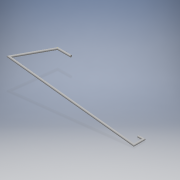
# Autodesk Inventor part: WIRE
Saved by Autodesk Inventor 2017 (Build 210142000, 142)
## iProperties
Created: 2017-12-26
Part Number: WIRE
Material: Generic
Document SubType Name: Modeling
Designer: will
Density: 1 g/cm^3
Appearance: Default
Author: will
Autodesk Inventor part; units mm, degrees
ref_plane "YZ Plane" through (0, 0, 0) normal (1, 0, 0) x (0, 1, 0)
ref_plane "XZ Plane" through (0, 0, 0) normal (0, 1, 0) x (-1, 0, 0)
ref_plane "XY Plane" through (0, 0, 0) normal (0, 0, 1) x (1, 0, 0)
sketch "Sketch1" plane through (0, 0, 0) normal (0, 0, 1) x (1, 0, 0)
  circle A0 centre (-10.0785, 9.8744) radius 0.8047
  point P0 (0, 0)
  constraints: 1 centre point
sketch3d "3D Sketch1"
  line L0 (-108.4342, 25.2423, -12.8177) -> (-113.0178, 25.2403, -13.7938)
  arc A0 (-113.0178, 25.2403, -13.7938) -> (-115.4344, 25.2393, -11.8377) centre (-113.4344, 25.2402, -11.8377) ccw
  line L1 (-115.4344, 25.2393, -11.8377) -> (-115.4344, 25.2393, 1.4693)
  arc A1 (-115.4344, 25.2393, 1.4693) -> (-113.4532, 24.9504, 3.4693) centre (-113.4554, 24.9507, 1.4693) ccw
  line L2 (-113.4532, 24.9504, 3.4693) -> (-12.0554, 10.1627, 3.3569)
  arc A2 (-12.0554, 10.1627, 3.3569) -> (-10.0785, 9.8744, 1.3569) centre (-12.0576, 10.163, 1.3569) ccw
  line L3 (-10.0785, 9.8744, 1.3569) -> (-10.0785, 9.8744, 0)
  line L4 (-10.0785, 9.8744, 0) -> (-10.0785, 9.8744, -2.8366)
  arc A3 (-10.0785, 9.8744, -2.8366) -> (-12.0785, 9.8744, -4.8366) centre (-12.0785, 9.8744, -2.8366) ccw
  line L5 (-12.0785, 9.8744, -4.8366) -> (-14.5001, 9.8744, -4.8366)
  dimension "d6" = 17.78
  dimension "d2" = 2
  dimension "d3" = 2
  dimension "d4" = 2
  dimension "d5" = 2
  constraints: 2 vertical, 6 other
sweep "Sweep1" add profiles "Sketch1" path "3D Sketch1"
equation "\"d3\" = d2"
equation "\"d4\" = d2"
equation "\"d5\" = d2"
body "Solid1"
